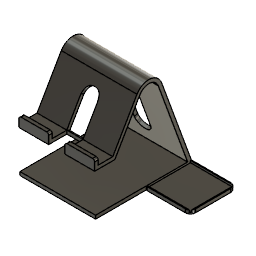
phone holder main (Autodesk Fusion 360 design; units mm, degrees)
part number: 2026-07-16-09-25-46-286
Autodesk Fusion 360 part; units mm, degrees
sketch "Sketch1" plane through (0, 0, 0) normal (1, 0, 0) x (0, 1, 0)
  line L0 (0, 0) -> (91.2113, 0)
  line L1 (91.2113, 0) -> (62.1396, 79.8739)
  line L2 (44.0824, 81.4537) -> (19.0824, 38.1524)
  line L3 (44.0824, 81.4537) -> (83.4301, 81.4537) construction
  line L4 (19.0824, 38.1524) -> (-0.9176, 38.1524)
  line L5 (-0.9176, 38.1524) -> (-0.9176, 48.1524)
  arc A0 (62.1396, 79.8739) -> (44.0824, 81.4537) centre (52.7426, 76.4537) ccw
  line L6 (0, -3.5) -> (96.2098, -3.5)
  line L7 (96.2098, -3.5) -> (65.4285, 81.0709)
  arc A1 (65.4285, 81.0709) -> (41.0513, 83.2037) centre (52.7426, 76.4537) ccw
  line L8 (41.0513, 83.2037) -> (17.0617, 41.6524)
  line L9 (17.0617, 41.6524) -> (2.5824, 41.6524)
  line L10 (2.5824, 41.6524) -> (2.5824, 48.1524)
  line L11 (-0.9176, 48.1524) -> (2.5824, 48.1524)
  line L12 (0, 0) -> (0, -3.5)
  dimension "d1" = 110
  dimension "d2" = 85
  dimension "d3" = 20
  dimension "d4" = 120
  dimension "d5" = 50
  dimension "d6" = 20
  dimension "d7" = 10
  dimension "d8" = 3.5
  constraint coincident L0.start L12.start
  constraint horizontal L0
  constraint tangent L1 A0
  constraint horizontal L3
  constraint tangent L2 A0
  constraint parallel L0 L4
  constraint perpendicular L4 L5
  constraint perpendicular L10 L11
  constraint perpendicular L6 L12
  measures "d1" angle of L0 L1
  measures "d2" distance of L0.end L1.end
  measures "d3" diameter of A0
  measures "d4" angle of L2 L3
  measures "d5" distance of L2.start L2.end
  measures "d6" distance of L2.end L4.end
  measures "d7" distance of L4.end L5.end
extrude "Extrude1" add sketch "Sketch1" along normal blind 75 makes body 1
sketch "Sketch2" plane through (0, 83.8305, 30.5118) normal (0, 0.939693, 0.34202) x (-1, 0, 0)
  line L0 (0, -36.1946) -> (0, 53.8039)
  line L1 (0, 53.8039) -> (-75, 53.8039)
  line L2 (-75, 53.8039) -> (-75, -36.1946)
  line L3 (-75, -36.1946) -> (0, -36.1946)
  line L4 (-45.5247, 21.2171) -> (-45.5247, -10)
  arc A0 (-45.5247, -10) -> (-29.4753, -10) centre (-37.5, -10) ccw
  line L5 (-29.4753, -10) -> (-29.4753, 21.2171)
  arc A1 (-29.4753, 21.2171) -> (-45.5247, 21.2171) centre (-37.5, 21.2171) ccw
  line L6 (-37.5, 21.2171) -> (-37.5, -10) construction
  constraint tangent L4 A0
  constraint tangent A0 L5
  constraint parallel L4 L5
  constraint tangent L5 A1
  constraint tangent L4 A1
  constraint perpendicular L1 L6
extrude "Extrude2" cut sketch "Sketch2" against normal blind 20 contours L4 A0 L5 A1 bodies 1
sketch "Sketch3" plane through (0, -0.9176, 0) normal (0, -1, 0) x (1, 0, 0)
  line L0 (0, 48.1524) -> (0, 38.1524)
  line L1 (0, 38.1524) -> (75, 38.1524)
  line L2 (75, 38.1524) -> (75, 48.1524)
  line L3 (75, 48.1524) -> (0, 48.1524)
  line L4 (0, 38.1524) -> (75, 38.1524)
  line L5 (0, 48.1524) -> (75, 48.1524)
  line L6 (29.4753, 19.9178) -> (29.4753, 49.2523)
  line L7 (45.5247, 49.2523) -> (45.5247, 19.9178)
  line L8 (29.4753, 38.1524) -> (45.5247, 38.1524)
  line L9 (45.5247, 38.1524) -> (45.5247, 48.1524)
  line L10 (45.5247, 48.1524) -> (29.4753, 48.1524)
  line L11 (29.4753, 48.1524) -> (29.4753, 38.1524)
  constraint horizontal L8
  constraint vertical L9
  constraint horizontal L10
  constraint vertical L11
  constraint coincident L5 L9.end
  constraint coincident L7 L9.end
  constraint coincident L6 L8.start
  constraint coincident L1 L8.start
extrude "Extrude3" cut sketch "Sketch3" against normal blind 18 contours L1 L3 L4 L5 L6 L7 L8 L9 L10 L11 bodies 1
sketch "Sketch4" plane through (0, -5.2398, 3.0252) normal (0, -0.866025, 0.5) x (1, 0, 0)
  line L0 (29.4753, 44.6029) -> (29.4753, 44.6443)
  line L1 (29.4753, 44.6443) -> (45.5247, 44.6443)
  line L2 (45.5247, 44.6443) -> (45.5247, 44.6029)
  line L3 (45.5247, 44.6029) -> (75, 44.6029)
  line L4 (75, 44.6029) -> (75, 92.5821)
  line L5 (75, 92.5821) -> (0, 92.5821)
  line L6 (0, 92.5821) -> (0, 44.6029)
  line L7 (0, 44.6029) -> (29.4753, 44.6029)
  line L8 (29.4753, 44.6029) -> (45.4753, 44.6029)
  line L9 (45.4753, 44.6029) -> (45.4753, 72.6029)
  line L10 (45.4753, 72.6029) -> (29.4753, 72.6029)
  line L11 (29.4753, 72.6029) -> (29.4753, 44.6029)
  spline S0 degree 5 poles (29.4753, 72.6029) (29.5205, 72.9235) (29.6212, 73.5517) (29.803, 74.4554) (30.107, 75.5825) (30.5901, 76.8606) (31.1758, 78.0057) (31.8619, 79.0155) (32.6433, 79.8874) (33.5114, 80.6188) (34.4528, 81.2077) (35.4502, 81.6536) (36.4834, 81.9576) (37.5303, 82.124) (38.5671, 82.1608) (39.57, 82.0807) (40.5161, 81.8977) (41.3866, 81.6235) (42.1676, 81.2645) (42.8534, 80.8178) (43.4458, 80.2716) (43.9509, 79.6104) (44.3764, 78.8182) (44.7293, 77.8835) (45.0145, 76.8) (45.2352, 75.5652) (45.3619, 74.4558) (45.4293, 73.5557) (45.462, 72.9255) (45.4753, 72.6029) knots 0 0 0 0 0 0 0.04 0.08 0.12 0.16 0.2 0.24 0.28 0.32 0.36 0.4 0.44 0.48 0.52 0.56 0.6 0.64 0.68 0.72 0.76 0.8 0.84 0.88 0.92 0.96 1 1 1 1 1 1
  point P0 (32.6462, 79.834)
  point P1 (37.4753, 82.0863)
  point P2 (41.7342, 81.4476)
  point P3 (44.1273, 79.2466)
  dimension "d15" = 16
  dimension "d16" = 28
  constraint horizontal L8
  constraint vertical L9
  constraint horizontal L10
  constraint vertical L11
  constraint coincident L0.start L7.end
  measures "d15" distance of L0.start L8.end
  measures "d16" distance of L0.start L10.end
extrude "Extrude4" cut sketch "Sketch4" against normal blind 5 contours L1 L9 L10 L11 | L10 S0 bodies 1
fillet "Fillet1" radius 2 1 edges at (75, 0.8324, 48.1524) on bodies 1
fillet "Fillet2" radius 2 1 edges at (45.5247, 0.8324, 48.1524) on bodies 1
fillet "Fillet3" radius 2 2 edges at (0, 0.8324, 48.1524) (29.4753, 0.8324, 48.1524) on bodies 1
sketch "Sketch5" plane through (0, 0, 0) normal (0, 0, 1) x (1, 0, 0)
  line L0 (74, 95) -> (119, 95)
  line L1 (119, 95) -> (119, 50)
  line L2 (119, 50) -> (74, 50)
  line L3 (74, 50) -> (74, 95)
  constraint horizontal L0
  constraint vertical L1
  constraint horizontal L2
  constraint vertical L3
extrude "Extrude5" add sketch "Sketch5" against normal blind 3.5 separate body makes body 2
sketch "Sketch6" plane through (0, 0, 0) normal (0, 0, 1) x (-1, 0, 0)
  line L0 (-74, -50) -> (-119, -50)
  line L1 (-119, -50) -> (-119, -95)
  line L2 (-119, -95) -> (-74, -95)
  line L3 (-74, -95) -> (-74, -50)
  line L4 (-75, -94) -> (-118, -94)
  line L5 (-118, -94) -> (-118, -51)
  line L6 (-118, -51) -> (-75, -51)
  line L7 (-75, -51) -> (-75, -94)
  constraint horizontal L4
  constraint vertical L5
  constraint horizontal L6
  constraint vertical L7
extrude "Extrude6" cut sketch "Sketch6" against normal blind 2 contours L4 L5 L6 L7 bodies 2
fillet "Fillet4" radius 5 1 edges at (119, 50, -1.75) on bodies 2
fillet "Fillet5" radius 5 1 edges at (119, 95, -1.75) on bodies 2
fillet "Fillet6" radius 2 1 edges at (74, 50, -1.75) on bodies 2
fillet "Fillet7" radius 2.5 1 edges at (74, 95, -1.75) on bodies 2
combine "Combine1" operation add target body 1 tool bodies 2
